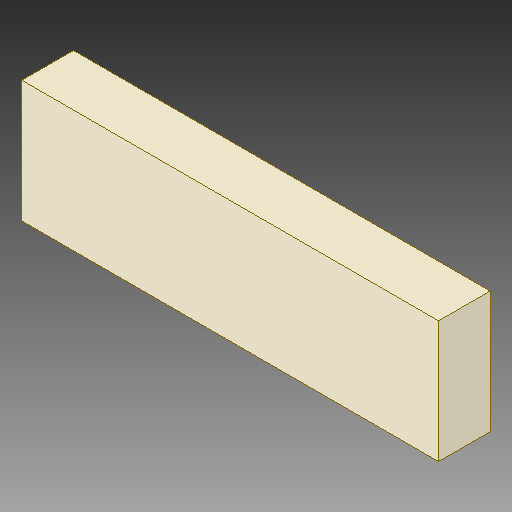
# Autodesk Inventor part: 10K
Saved by Autodesk Inventor 2017 (Build 210142000, 142)
## iProperties
Created: 2019-06-13
Part Number: 10K
Material: Generic
Document SubType Name: Modeling
Designer: Marc
Density: 1 g/cm^3
Appearance: 0207_9, 10K
Author: Marc
Autodesk Inventor part; units mm, degrees
ref_plane "YZ Plane" through (0, 0, 0) normal (1, 0, 0) x (0, 1, 0)
ref_plane "XZ Plane" through (0, 0, 0) normal (0, 1, 0) x (-1, 0, 0)
ref_plane "XY Plane" through (0, 0, 0) normal (0, 0, 1) x (1, 0, 0)
sketch "0207_9, 10K_50" plane through (0, 0, 0) normal (0, 0, 1) x (1, 0, 0)
  line L0 (-4.0386, 1.2192) -> (4.0386, 1.2192)
  line L1 (4.0386, 1.2192) -> (4.0386, -1.143)
  line L2 (4.0386, -1.143) -> (-4.0386, -1.143)
  line L3 (-4.0386, -1.143) -> (-4.0386, 1.2192)
  constraints: 8 end point
extrude "Extrusion1" add sketch "0207_9, 10K_50" along normal blind 1
body "Solid1"
